Autodesk Fusion 360 part; units mm, degrees
note: some values were not read from the file. Chosen so that the rebuilt part matches the saved one: which bodies a step acts on.
(part 3 of 5)
sketch "スケッチ1 (13)" plane through (0, 0, 0) normal (0, 0, 1) x (1, 0, 0) in component "Stage2_Sun_Gear"
  line L0 (13.0702, -1.1985) -> (14.0365, -1.2871)
  line L1 (14.0365, -1.2871) -> (14.8505, -1.1753)
  line L2 (14.8505, -1.1753) -> (15.673, -0.8944)
  line L3 (15.673, -0.8944) -> (16.4928, -0.4881)
  line L4 (16.4928, -0.4881) -> (16.4928, 0.4881)
  line L5 (16.4928, 0.4881) -> (15.673, 0.8944)
  line L6 (15.673, 0.8944) -> (14.8505, 1.1753)
  line L7 (14.8505, 1.1753) -> (14.0365, 1.2871)
  line L8 (14.0365, 1.2871) -> (13.0702, 1.1985)
  line L9 (13.0702, 1.1985) -> (12.9634, 2.0532)
  line L10 (12.9634, 2.0532) -> (12.8008, 2.899)
  line L11 (12.8008, 2.899) -> (13.7473, 3.1134)
  line L12 (13.7473, 3.1134) -> (14.4868, 3.4713)
  line L13 (14.4868, 3.4713) -> (15.1822, 3.9926)
  line L14 (15.1822, 3.9926) -> (15.8364, 4.6323)
  line L15 (15.8364, 4.6323) -> (15.5347, 5.5607)
  line L16 (15.5347, 5.5607) -> (14.6295, 5.6938)
  line L17 (14.6295, 5.6938) -> (13.7605, 5.7068)
  line L18 (13.7605, 5.7068) -> (12.9518, 5.5617)
  line L19 (12.9518, 5.5617) -> (12.0601, 5.1788)
  line L20 (12.0601, 5.1788) -> (11.6945, 5.9586)
  line L21 (11.6945, 5.9586) -> (11.2785, 6.7128)
  line L22 (11.2785, 6.7128) -> (12.1123, 7.2091)
  line L23 (12.1123, 7.2091) -> (12.7051, 7.7781)
  line L24 (12.7051, 7.7781) -> (13.2054, 8.4888)
  line L25 (13.2054, 8.4888) -> (13.6298, 9.2993)
  line L26 (13.6298, 9.2993) -> (13.056, 10.0891)
  line L27 (13.056, 10.0891) -> (12.154, 9.9359)
  line L28 (12.154, 9.9359) -> (11.3235, 9.6797)
  line L29 (11.3235, 9.6797) -> (10.5992, 9.2918)
  line L30 (10.5992, 9.2918) -> (9.8695, 8.6521)
  line L31 (9.8695, 8.6521) -> (9.2808, 9.2808)
  line L32 (9.2808, 9.2808) -> (8.6521, 9.8695)
  line L33 (8.6521, 9.8695) -> (9.2918, 10.5992)
  line L34 (9.2918, 10.5992) -> (9.6797, 11.3235)
  line L35 (9.6797, 11.3235) -> (9.9359, 12.154)
  line L36 (9.9359, 12.154) -> (10.0891, 13.056)
  line L37 (10.0891, 13.056) -> (9.2993, 13.6298)
  line L38 (9.2993, 13.6298) -> (8.4888, 13.2054)
  line L39 (8.4888, 13.2054) -> (7.7781, 12.7051)
  line L40 (7.7781, 12.7051) -> (7.2091, 12.1123)
  line L41 (7.2091, 12.1123) -> (6.7128, 11.2785)
  line L42 (6.7128, 11.2785) -> (5.9586, 11.6945)
  line L43 (5.9586, 11.6945) -> (5.1788, 12.0601)
  line L44 (5.1788, 12.0601) -> (5.5617, 12.9518)
  line L45 (5.5617, 12.9518) -> (5.7068, 13.7605)
  line L46 (5.7068, 13.7605) -> (5.6938, 14.6295)
  line L47 (5.6938, 14.6295) -> (5.5607, 15.5347)
  line L48 (5.5607, 15.5347) -> (4.6323, 15.8364)
  line L49 (4.6323, 15.8364) -> (3.9926, 15.1822)
  line L50 (3.9926, 15.1822) -> (3.4713, 14.4868)
  line L51 (3.4713, 14.4868) -> (3.1134, 13.7473)
  line L52 (3.1134, 13.7473) -> (2.899, 12.8008)
  line L53 (2.899, 12.8008) -> (2.0532, 12.9634)
  line L54 (2.0532, 12.9634) -> (1.1985, 13.0702)
  line L55 (1.1985, 13.0702) -> (1.2871, 14.0365)
  line L56 (1.2871, 14.0365) -> (1.1753, 14.8505)
  line L57 (1.1753, 14.8505) -> (0.8944, 15.673)
  line L58 (0.8944, 15.673) -> (0.4881, 16.4928)
  line L59 (0.4881, 16.4928) -> (-0.4881, 16.4928)
  line L60 (-0.4881, 16.4928) -> (-0.8944, 15.673)
  line L61 (-0.8944, 15.673) -> (-1.1753, 14.8505)
  line L62 (-1.1753, 14.8505) -> (-1.2871, 14.0365)
  line L63 (-1.2871, 14.0365) -> (-1.1985, 13.0702)
  line L64 (-1.1985, 13.0702) -> (-2.0532, 12.9634)
  line L65 (-2.0532, 12.9634) -> (-2.899, 12.8008)
  line L66 (-2.899, 12.8008) -> (-3.1134, 13.7473)
  line L67 (-3.1134, 13.7473) -> (-3.4713, 14.4868)
  line L68 (-3.4713, 14.4868) -> (-3.9926, 15.1822)
  line L69 (-3.9926, 15.1822) -> (-4.6323, 15.8364)
  line L70 (-4.6323, 15.8364) -> (-5.5607, 15.5347)
  line L71 (-5.5607, 15.5347) -> (-5.6938, 14.6295)
  line L72 (-5.6938, 14.6295) -> (-5.7068, 13.7605)
  line L73 (-5.7068, 13.7605) -> (-5.5617, 12.9518)
  line L74 (-5.5617, 12.9518) -> (-5.1788, 12.0601)
  line L75 (-5.1788, 12.0601) -> (-5.9586, 11.6945)
  line L76 (-5.9586, 11.6945) -> (-6.7128, 11.2785)
  line L77 (-6.7128, 11.2785) -> (-7.2091, 12.1123)
  line L78 (-7.2091, 12.1123) -> (-7.7781, 12.7051)
  line L79 (-7.7781, 12.7051) -> (-8.4888, 13.2054)
  line L80 (-8.4888, 13.2054) -> (-9.2993, 13.6298)
  line L81 (-9.2993, 13.6298) -> (-10.0891, 13.056)
  line L82 (-10.0891, 13.056) -> (-9.9359, 12.154)
  line L83 (-9.9359, 12.154) -> (-9.6797, 11.3235)
  line L84 (-9.6797, 11.3235) -> (-9.2918, 10.5992)
  line L85 (-9.2918, 10.5992) -> (-8.6521, 9.8695)
  line L86 (-8.6521, 9.8695) -> (-9.2808, 9.2808)
  line L87 (-9.2808, 9.2808) -> (-9.8695, 8.6521)
  line L88 (-9.8695, 8.6521) -> (-10.5992, 9.2918)
  line L89 (-10.5992, 9.2918) -> (-11.3235, 9.6797)
  line L90 (-11.3235, 9.6797) -> (-12.154, 9.9359)
  line L91 (-12.154, 9.9359) -> (-13.056, 10.0891)
  line L92 (-13.056, 10.0891) -> (-13.6298, 9.2993)
  line L93 (-13.6298, 9.2993) -> (-13.2054, 8.4888)
  line L94 (-13.2054, 8.4888) -> (-12.7051, 7.7781)
  line L95 (-12.7051, 7.7781) -> (-12.1123, 7.2091)
  line L96 (-12.1123, 7.2091) -> (-11.2785, 6.7128)
  line L97 (-11.2785, 6.7128) -> (-11.6945, 5.9586)
  line L98 (-11.6945, 5.9586) -> (-12.0601, 5.1788)
  line L99 (-12.0601, 5.1788) -> (-12.9518, 5.5617)
  line L100 (-12.9518, 5.5617) -> (-13.7605, 5.7068)
  line L101 (-13.7605, 5.7068) -> (-14.6295, 5.6938)
  line L102 (-14.6295, 5.6938) -> (-15.5347, 5.5607)
  line L103 (-15.5347, 5.5607) -> (-15.8364, 4.6323)
  line L104 (-15.8364, 4.6323) -> (-15.1822, 3.9926)
  line L105 (-15.1822, 3.9926) -> (-14.4868, 3.4713)
  line L106 (-14.4868, 3.4713) -> (-13.7473, 3.1134)
  line L107 (-13.7473, 3.1134) -> (-12.8008, 2.899)
  line L108 (-12.8008, 2.899) -> (-12.9634, 2.0532)
  line L109 (-12.9634, 2.0532) -> (-13.0702, 1.1985)
  line L110 (-13.0702, 1.1985) -> (-14.0365, 1.2871)
  line L111 (-14.0365, 1.2871) -> (-14.8505, 1.1753)
  line L112 (-14.8505, 1.1753) -> (-15.673, 0.8944)
  line L113 (-15.673, 0.8944) -> (-16.4928, 0.4881)
  line L114 (-16.4928, 0.4881) -> (-16.4928, -0.4881)
  line L115 (-16.4928, -0.4881) -> (-15.673, -0.8944)
  line L116 (-15.673, -0.8944) -> (-14.8505, -1.1753)
  line L117 (-14.8505, -1.1753) -> (-14.0365, -1.2871)
  line L118 (-14.0365, -1.2871) -> (-13.0702, -1.1985)
  line L119 (-13.0702, -1.1985) -> (-12.9634, -2.0532)
  line L120 (-12.9634, -2.0532) -> (-12.8008, -2.899)
  line L121 (-12.8008, -2.899) -> (-13.7473, -3.1134)
  line L122 (-13.7473, -3.1134) -> (-14.4868, -3.4713)
  line L123 (-14.4868, -3.4713) -> (-15.1822, -3.9926)
  line L124 (-15.1822, -3.9926) -> (-15.8364, -4.6323)
  line L125 (-15.8364, -4.6323) -> (-15.5347, -5.5607)
  line L126 (-15.5347, -5.5607) -> (-14.6295, -5.6938)
  line L127 (-14.6295, -5.6938) -> (-13.7605, -5.7068)
  line L128 (-13.7605, -5.7068) -> (-12.9518, -5.5617)
  line L129 (-12.9518, -5.5617) -> (-12.0601, -5.1788)
  line L130 (-12.0601, -5.1788) -> (-11.6945, -5.9586)
  line L131 (-11.6945, -5.9586) -> (-11.2785, -6.7128)
  line L132 (-11.2785, -6.7128) -> (-12.1123, -7.2091)
  line L133 (-12.1123, -7.2091) -> (-12.7051, -7.7781)
  line L134 (-12.7051, -7.7781) -> (-13.2054, -8.4888)
  line L135 (-13.2054, -8.4888) -> (-13.6298, -9.2993)
  line L136 (-13.6298, -9.2993) -> (-13.056, -10.0891)
  line L137 (-13.056, -10.0891) -> (-12.154, -9.9359)
  line L138 (-12.154, -9.9359) -> (-11.3235, -9.6797)
  line L139 (-11.3235, -9.6797) -> (-10.5992, -9.2918)
  line L140 (-10.5992, -9.2918) -> (-9.8695, -8.6521)
  line L141 (-9.8695, -8.6521) -> (-9.2808, -9.2808)
  line L142 (-9.2808, -9.2808) -> (-8.6521, -9.8695)
  line L143 (-8.6521, -9.8695) -> (-9.2918, -10.5992)
  line L144 (-9.2918, -10.5992) -> (-9.6797, -11.3235)
  line L145 (-9.6797, -11.3235) -> (-9.9359, -12.154)
  line L146 (-9.9359, -12.154) -> (-10.0891, -13.056)
  line L147 (-10.0891, -13.056) -> (-9.2993, -13.6298)
  line L148 (-9.2993, -13.6298) -> (-8.4888, -13.2054)
  line L149 (-8.4888, -13.2054) -> (-7.7781, -12.7051)
  line L150 (-7.7781, -12.7051) -> (-7.2091, -12.1123)
  line L151 (-7.2091, -12.1123) -> (-6.7128, -11.2785)
  line L152 (-6.7128, -11.2785) -> (-5.9586, -11.6945)
  line L153 (-5.9586, -11.6945) -> (-5.1788, -12.0601)
  line L154 (-5.1788, -12.0601) -> (-5.5617, -12.9518)
  line L155 (-5.5617, -12.9518) -> (-5.7068, -13.7605)
  line L156 (-5.7068, -13.7605) -> (-5.6938, -14.6295)
  line L157 (-5.6938, -14.6295) -> (-5.5607, -15.5347)
  line L158 (-5.5607, -15.5347) -> (-4.6323, -15.8364)
  line L159 (-4.6323, -15.8364) -> (-3.9926, -15.1822)
  line L160 (-3.9926, -15.1822) -> (-3.4713, -14.4868)
  line L161 (-3.4713, -14.4868) -> (-3.1134, -13.7473)
  line L162 (-3.1134, -13.7473) -> (-2.899, -12.8008)
  line L163 (-2.899, -12.8008) -> (-2.0532, -12.9634)
  line L164 (-2.0532, -12.9634) -> (-1.1985, -13.0702)
  line L165 (-1.1985, -13.0702) -> (-1.2871, -14.0365)
  line L166 (-1.2871, -14.0365) -> (-1.1753, -14.8505)
  line L167 (-1.1753, -14.8505) -> (-0.8944, -15.673)
  line L168 (-0.8944, -15.673) -> (-0.4881, -16.4928)
  line L169 (-0.4881, -16.4928) -> (0.4881, -16.4928)
  line L170 (0.4881, -16.4928) -> (0.8944, -15.673)
  line L171 (0.8944, -15.673) -> (1.1753, -14.8505)
  line L172 (1.1753, -14.8505) -> (1.2871, -14.0365)
  line L173 (1.2871, -14.0365) -> (1.1985, -13.0702)
  line L174 (1.1985, -13.0702) -> (2.0532, -12.9634)
  line L175 (2.0532, -12.9634) -> (2.899, -12.8008)
  line L176 (2.899, -12.8008) -> (3.1134, -13.7473)
  line L177 (3.1134, -13.7473) -> (3.4713, -14.4868)
  line L178 (3.4713, -14.4868) -> (3.9926, -15.1822)
  line L179 (3.9926, -15.1822) -> (4.6323, -15.8364)
  line L180 (4.6323, -15.8364) -> (5.5607, -15.5347)
  line L181 (5.5607, -15.5347) -> (5.6938, -14.6295)
  line L182 (5.6938, -14.6295) -> (5.7068, -13.7605)
  line L183 (5.7068, -13.7605) -> (5.5617, -12.9518)
  line L184 (5.5617, -12.9518) -> (5.1788, -12.0601)
  line L185 (5.1788, -12.0601) -> (5.9586, -11.6945)
  line L186 (5.9586, -11.6945) -> (6.7128, -11.2785)
  line L187 (6.7128, -11.2785) -> (7.2091, -12.1123)
  line L188 (7.2091, -12.1123) -> (7.7781, -12.7051)
  line L189 (7.7781, -12.7051) -> (8.4888, -13.2054)
  line L190 (8.4888, -13.2054) -> (9.2993, -13.6298)
  line L191 (9.2993, -13.6298) -> (10.0891, -13.056)
  line L192 (10.0891, -13.056) -> (9.9359, -12.154)
  line L193 (9.9359, -12.154) -> (9.6797, -11.3235)
  line L194 (9.6797, -11.3235) -> (9.2918, -10.5992)
  line L195 (9.2918, -10.5992) -> (8.6521, -9.8695)
  line L196 (8.6521, -9.8695) -> (9.2808, -9.2808)
  line L197 (9.2808, -9.2808) -> (9.8695, -8.6521)
  line L198 (9.8695, -8.6521) -> (10.5992, -9.2918)
  line L199 (10.5992, -9.2918) -> (11.3235, -9.6797)
  line L200 (11.3235, -9.6797) -> (12.154, -9.9359)
  line L201 (12.154, -9.9359) -> (13.056, -10.0891)
  line L202 (13.056, -10.0891) -> (13.6298, -9.2993)
  line L203 (13.6298, -9.2993) -> (13.2054, -8.4888)
  line L204 (13.2054, -8.4888) -> (12.7051, -7.7781)
  line L205 (12.7051, -7.7781) -> (12.1123, -7.2091)
  line L206 (12.1123, -7.2091) -> (11.2785, -6.7128)
  line L207 (11.2785, -6.7128) -> (11.6945, -5.9586)
  line L208 (11.6945, -5.9586) -> (12.0601, -5.1788)
  line L209 (12.0601, -5.1788) -> (12.9518, -5.5617)
  line L210 (12.9518, -5.5617) -> (13.7605, -5.7068)
  line L211 (13.7605, -5.7068) -> (14.6295, -5.6938)
  line L212 (14.6295, -5.6938) -> (15.5347, -5.5607)
  line L213 (15.5347, -5.5607) -> (15.8364, -4.6323)
  line L214 (15.8364, -4.6323) -> (15.1822, -3.9926)
  line L215 (15.1822, -3.9926) -> (14.4868, -3.4713)
  line L216 (14.4868, -3.4713) -> (13.7473, -3.1134)
  line L217 (13.7473, -3.1134) -> (12.8008, -2.899)
  line L218 (12.8008, -2.899) -> (12.9634, -2.0532)
  line L219 (12.9634, -2.0532) -> (13.0702, -1.1985)
extrude "Stage2_Sun_Extrude" add sketch "スケッチ1 (13)" along normal blind 12 from surface at 74 separate body makes body 14 in component "Stage2_Sun_Gear"
sketch "スケッチ2 (13)" plane through (0, 0, 0) normal (0, 0, 1) x (1, 0, 0) in component "Stage2_Sun_Gear"
  circle A0 centre (0, 0) radius 12
extrude "Stage2_Sun_Hub_Lower_Extrude" add sketch "スケッチ2 (13)" along normal blind 3 from surface at 71 bodies 14 in component "Stage2_Sun_Gear"
sketch "スケッチ3 (12)" plane through (0, 0, 0) normal (0, 0, 1) x (1, 0, 0) in component "Stage2_Sun_Gear"
  circle A0 centre (0, 0) radius 12
extrude "Stage2_Sun_Hub_Upper_Extrude" add sketch "スケッチ3 (12)" along normal blind 3 from surface at 86 bodies 14 in component "Stage2_Sun_Gear"
sketch "スケッチ4 (12)" plane through (0, 0, 0) normal (0, 0, 1) x (1, 0, 0) in component "Stage2_Sun_Gear"
  circle A0 centre (0, 0) radius 8.1
extrude "Stage2_Sun_Bore_Cut" cut sketch "スケッチ4 (12)" along normal blind 20 from surface at 70 bodies 14 in component "Stage2_Sun_Gear"
sketch "スケッチ1 (14)" plane through (0, 0, 0) normal (0, 0, 1) x (1, 0, 0) in component "Stage2_Planet_Gear_A"
  line L0 (17.2782, 3.2284) -> (16.3377, 3.4671)
  line L1 (16.3377, 3.4671) -> (15.5162, 3.4839)
  line L2 (15.5162, 3.4839) -> (14.6599, 3.3351)
  line L3 (14.6599, 3.3351) -> (13.7866, 3.0621)
  line L4 (13.7866, 3.0621) -> (13.6339, 2.098)
  line L5 (13.6339, 2.098) -> (14.3801, 1.5685)
  line L6 (14.3801, 1.5685) -> (15.1485, 1.1623)
  line L7 (15.1485, 1.1623) -> (15.935, 0.9245)
  line L8 (15.935, 0.9245) -> (16.9033, 0.8608)
  line L9 (16.9033, 0.8608) -> (16.875, 0)
  line L10 (16.875, 0) -> (16.9033, -0.8608)
  line L11 (16.9033, -0.8608) -> (15.935, -0.9245)
  line L12 (15.935, -0.9245) -> (15.1485, -1.1623)
  line L13 (15.1485, -1.1623) -> (14.3801, -1.5685)
  line L14 (14.3801, -1.5685) -> (13.6339, -2.098)
  line L15 (13.6339, -2.098) -> (13.7866, -3.0621)
  line L16 (13.7866, -3.0621) -> (14.6599, -3.3351)
  line L17 (14.6599, -3.3351) -> (15.5162, -3.4839)
  line L18 (15.5162, -3.4839) -> (16.3377, -3.4671)
  line L19 (16.3377, -3.4671) -> (17.2782, -3.2284)
  line L20 (17.2782, -3.2284) -> (17.5174, -4.0558)
  line L21 (17.5174, -4.0558) -> (17.8103, -4.8658)
  line L22 (17.8103, -4.8658) -> (16.909, -5.2256)
  line L23 (16.909, -5.2256) -> (16.2346, -5.6948)
  line L24 (16.2346, -5.6948) -> (15.6293, -6.3185)
  line L25 (15.6293, -6.3185) -> (15.0832, -7.0527)
  line L26 (15.0832, -7.0527) -> (15.5264, -7.9225)
  line L27 (15.5264, -7.9225) -> (16.4413, -7.9123)
  line L28 (16.4413, -7.9123) -> (17.3017, -7.7891)
  line L29 (17.3017, -7.7891) -> (18.0777, -7.5193)
  line L30 (18.0777, -7.5193) -> (18.8985, -7.0016)
  line L31 (18.8985, -7.0016) -> (19.3817, -7.7147)
  line L32 (19.3817, -7.7147) -> (19.9105, -8.3945)
  line L33 (19.9105, -8.3945) -> (19.1645, -9.0152)
  line L34 (19.1645, -9.0152) -> (18.6681, -9.6699)
  line L35 (18.6681, -9.6699) -> (18.2851, -10.4501)
  line L36 (18.2851, -10.4501) -> (17.9927, -11.317)
  line L37 (17.9927, -11.317) -> (18.683, -12.0073)
  line L38 (18.683, -12.0073) -> (19.5499, -11.7149)
  line L39 (19.5499, -11.7149) -> (20.3301, -11.3319)
  line L40 (20.3301, -11.3319) -> (20.9848, -10.8355)
  line L41 (20.9848, -10.8355) -> (21.6055, -10.0895)
  line L42 (21.6055, -10.0895) -> (22.2853, -10.6183)
  line L43 (22.2853, -10.6183) -> (22.9984, -11.1015)
  line L44 (22.9984, -11.1015) -> (22.4807, -11.9223)
  line L45 (22.4807, -11.9223) -> (22.2109, -12.6983)
  line L46 (22.2109, -12.6983) -> (22.0877, -13.5587)
  line L47 (22.0877, -13.5587) -> (22.0775, -14.4736)
  line L48 (22.0775, -14.4736) -> (22.9473, -14.9168)
  line L49 (22.9473, -14.9168) -> (23.6815, -14.3707)
  line L50 (23.6815, -14.3707) -> (24.3052, -13.7654)
  line L51 (24.3052, -13.7654) -> (24.7744, -13.091)
  line L52 (24.7744, -13.091) -> (25.1342, -12.1897)
  line L53 (25.1342, -12.1897) -> (25.9442, -12.4826)
  line L54 (25.9442, -12.4826) -> (26.7716, -12.7218)
  line L55 (26.7716, -12.7218) -> (26.5329, -13.6623)
  line L56 (26.5329, -13.6623) -> (26.5161, -14.4838)
  line L57 (26.5161, -14.4838) -> (26.6649, -15.3401)
  line L58 (26.6649, -15.3401) -> (26.9379, -16.2134)
  line L59 (26.9379, -16.2134) -> (27.902, -16.3661)
  line L60 (27.902, -16.3661) -> (28.4315, -15.6199)
  line L61 (28.4315, -15.6199) -> (28.8377, -14.8515)
  line L62 (28.8377, -14.8515) -> (29.0755, -14.065)
  line L63 (29.0755, -14.065) -> (29.1392, -13.0967)
  line L64 (29.1392, -13.0967) -> (30, -13.125)
  line L65 (30, -13.125) -> (30.8608, -13.0967)
  line L66 (30.8608, -13.0967) -> (30.9245, -14.065)
  line L67 (30.9245, -14.065) -> (31.1623, -14.8515)
  line L68 (31.1623, -14.8515) -> (31.5685, -15.6199)
  line L69 (31.5685, -15.6199) -> (32.098, -16.3661)
  line L70 (32.098, -16.3661) -> (33.0621, -16.2134)
  line L71 (33.0621, -16.2134) -> (33.3351, -15.3401)
  line L72 (33.3351, -15.3401) -> (33.4839, -14.4838)
  line L73 (33.4839, -14.4838) -> (33.4671, -13.6623)
  line L74 (33.4671, -13.6623) -> (33.2284, -12.7218)
  line L75 (33.2284, -12.7218) -> (34.0558, -12.4826)
  line L76 (34.0558, -12.4826) -> (34.8658, -12.1897)
  line L77 (34.8658, -12.1897) -> (35.2256, -13.091)
  line L78 (35.2256, -13.091) -> (35.6948, -13.7654)
  line L79 (35.6948, -13.7654) -> (36.3185, -14.3707)
  line L80 (36.3185, -14.3707) -> (37.0527, -14.9168)
  line L81 (37.0527, -14.9168) -> (37.9225, -14.4736)
  line L82 (37.9225, -14.4736) -> (37.9123, -13.5587)
  line L83 (37.9123, -13.5587) -> (37.7891, -12.6983)
  line L84 (37.7891, -12.6983) -> (37.5193, -11.9223)
  line L85 (37.5193, -11.9223) -> (37.0016, -11.1015)
  line L86 (37.0016, -11.1015) -> (37.7147, -10.6183)
  line L87 (37.7147, -10.6183) -> (38.3945, -10.0895)
  line L88 (38.3945, -10.0895) -> (39.0152, -10.8355)
  line L89 (39.0152, -10.8355) -> (39.6699, -11.3319)
  line L90 (39.6699, -11.3319) -> (40.4501, -11.7149)
  line L91 (40.4501, -11.7149) -> (41.317, -12.0073)
  line L92 (41.317, -12.0073) -> (42.0073, -11.317)
  line L93 (42.0073, -11.317) -> (41.7149, -10.4501)
  line L94 (41.7149, -10.4501) -> (41.3319, -9.6699)
  line L95 (41.3319, -9.6699) -> (40.8355, -9.0152)
  line L96 (40.8355, -9.0152) -> (40.0895, -8.3945)
  line L97 (40.0895, -8.3945) -> (40.6183, -7.7147)
  line L98 (40.6183, -7.7147) -> (41.1015, -7.0016)
  line L99 (41.1015, -7.0016) -> (41.9223, -7.5193)
  line L100 (41.9223, -7.5193) -> (42.6983, -7.7891)
  line L101 (42.6983, -7.7891) -> (43.5587, -7.9123)
  line L102 (43.5587, -7.9123) -> (44.4736, -7.9225)
  line L103 (44.4736, -7.9225) -> (44.9168, -7.0527)
  line L104 (44.9168, -7.0527) -> (44.3707, -6.3185)
  line L105 (44.3707, -6.3185) -> (43.7654, -5.6948)
  line L106 (43.7654, -5.6948) -> (43.091, -5.2256)
  line L107 (43.091, -5.2256) -> (42.1897, -4.8658)
  line L108 (42.1897, -4.8658) -> (42.4826, -4.0558)
  line L109 (42.4826, -4.0558) -> (42.7218, -3.2284)
  line L110 (42.7218, -3.2284) -> (43.6623, -3.4671)
  line L111 (43.6623, -3.4671) -> (44.4838, -3.4839)
  line L112 (44.4838, -3.4839) -> (45.3401, -3.3351)
  line L113 (45.3401, -3.3351) -> (46.2134, -3.0621)
  line L114 (46.2134, -3.0621) -> (46.3661, -2.098)
  line L115 (46.3661, -2.098) -> (45.6199, -1.5685)
  line L116 (45.6199, -1.5685) -> (44.8515, -1.1623)
  line L117 (44.8515, -1.1623) -> (44.065, -0.9245)
  line L118 (44.065, -0.9245) -> (43.0967, -0.8608)
  line L119 (43.0967, -0.8608) -> (43.125, 0)
  line L120 (43.125, 0) -> (43.0967, 0.8608)
  line L121 (43.0967, 0.8608) -> (44.065, 0.9245)
  line L122 (44.065, 0.9245) -> (44.8515, 1.1623)
  line L123 (44.8515, 1.1623) -> (45.6199, 1.5685)
  line L124 (45.6199, 1.5685) -> (46.3661, 2.098)
  line L125 (46.3661, 2.098) -> (46.2134, 3.0621)
  line L126 (46.2134, 3.0621) -> (45.3401, 3.3351)
  line L127 (45.3401, 3.3351) -> (44.4838, 3.4839)
  line L128 (44.4838, 3.4839) -> (43.6623, 3.4671)
  line L129 (43.6623, 3.4671) -> (42.7218, 3.2284)
  line L130 (42.7218, 3.2284) -> (42.4826, 4.0558)
  line L131 (42.4826, 4.0558) -> (42.1897, 4.8658)
  line L132 (42.1897, 4.8658) -> (43.091, 5.2256)
  line L133 (43.091, 5.2256) -> (43.7654, 5.6948)
  line L134 (43.7654, 5.6948) -> (44.3707, 6.3185)
  line L135 (44.3707, 6.3185) -> (44.9168, 7.0527)
  line L136 (44.9168, 7.0527) -> (44.4736, 7.9225)
  line L137 (44.4736, 7.9225) -> (43.5587, 7.9123)
  line L138 (43.5587, 7.9123) -> (42.6983, 7.7891)
  line L139 (42.6983, 7.7891) -> (41.9223, 7.5193)
  line L140 (41.9223, 7.5193) -> (41.1015, 7.0016)
  line L141 (41.1015, 7.0016) -> (40.6183, 7.7147)
  line L142 (40.6183, 7.7147) -> (40.0895, 8.3945)
  line L143 (40.0895, 8.3945) -> (40.8355, 9.0152)
  line L144 (40.8355, 9.0152) -> (41.3319, 9.6699)
  line L145 (41.3319, 9.6699) -> (41.7149, 10.4501)
  line L146 (41.7149, 10.4501) -> (42.0073, 11.317)
  line L147 (42.0073, 11.317) -> (41.317, 12.0073)
  line L148 (41.317, 12.0073) -> (40.4501, 11.7149)
  line L149 (40.4501, 11.7149) -> (39.6699, 11.3319)
  line L150 (39.6699, 11.3319) -> (39.0152, 10.8355)
  line L151 (39.0152, 10.8355) -> (38.3945, 10.0895)
  line L152 (38.3945, 10.0895) -> (37.7147, 10.6183)
  line L153 (37.7147, 10.6183) -> (37.0016, 11.1015)
  line L154 (37.0016, 11.1015) -> (37.5193, 11.9223)
  line L155 (37.5193, 11.9223) -> (37.7891, 12.6983)
  line L156 (37.7891, 12.6983) -> (37.9123, 13.5587)
  line L157 (37.9123, 13.5587) -> (37.9225, 14.4736)
  line L158 (37.9225, 14.4736) -> (37.0527, 14.9168)
  line L159 (37.0527, 14.9168) -> (36.3185, 14.3707)
  line L160 (36.3185, 14.3707) -> (35.6948, 13.7654)
  line L161 (35.6948, 13.7654) -> (35.2256, 13.091)
  line L162 (35.2256, 13.091) -> (34.8658, 12.1897)
  line L163 (34.8658, 12.1897) -> (34.0558, 12.4826)
  line L164 (34.0558, 12.4826) -> (33.2284, 12.7218)
  line L165 (33.2284, 12.7218) -> (33.4671, 13.6623)
  line L166 (33.4671, 13.6623) -> (33.4839, 14.4838)
  line L167 (33.4839, 14.4838) -> (33.3351, 15.3401)
  line L168 (33.3351, 15.3401) -> (33.0621, 16.2134)
  line L169 (33.0621, 16.2134) -> (32.098, 16.3661)
  line L170 (32.098, 16.3661) -> (31.5685, 15.6199)
  line L171 (31.5685, 15.6199) -> (31.1623, 14.8515)
  line L172 (31.1623, 14.8515) -> (30.9245, 14.065)
  line L173 (30.9245, 14.065) -> (30.8608, 13.0967)
  line L174 (30.8608, 13.0967) -> (30, 13.125)
  line L175 (30, 13.125) -> (29.1392, 13.0967)
  line L176 (29.1392, 13.0967) -> (29.0755, 14.065)
  line L177 (29.0755, 14.065) -> (28.8377, 14.8515)
  line L178 (28.8377, 14.8515) -> (28.4315, 15.6199)
  line L179 (28.4315, 15.6199) -> (27.902, 16.3661)
  line L180 (27.902, 16.3661) -> (26.9379, 16.2134)
  line L181 (26.9379, 16.2134) -> (26.6649, 15.3401)
  line L182 (26.6649, 15.3401) -> (26.5161, 14.4838)
  line L183 (26.5161, 14.4838) -> (26.5329, 13.6623)
  line L184 (26.5329, 13.6623) -> (26.7716, 12.7218)
  line L185 (26.7716, 12.7218) -> (25.9442, 12.4826)
  line L186 (25.9442, 12.4826) -> (25.1342, 12.1897)
  line L187 (25.1342, 12.1897) -> (24.7744, 13.091)
  line L188 (24.7744, 13.091) -> (24.3052, 13.7654)
  line L189 (24.3052, 13.7654) -> (23.6815, 14.3707)
  line L190 (23.6815, 14.3707) -> (22.9473, 14.9168)
  line L191 (22.9473, 14.9168) -> (22.0775, 14.4736)
  line L192 (22.0775, 14.4736) -> (22.0877, 13.5587)
  line L193 (22.0877, 13.5587) -> (22.2109, 12.6983)
  line L194 (22.2109, 12.6983) -> (22.4807, 11.9223)
  line L195 (22.4807, 11.9223) -> (22.9984, 11.1015)
  line L196 (22.9984, 11.1015) -> (22.2853, 10.6183)
  line L197 (22.2853, 10.6183) -> (21.6055, 10.0895)
  line L198 (21.6055, 10.0895) -> (20.9848, 10.8355)
  line L199 (20.9848, 10.8355) -> (20.3301, 11.3319)
  line L200 (20.3301, 11.3319) -> (19.5499, 11.7149)
  line L201 (19.5499, 11.7149) -> (18.683, 12.0073)
  line L202 (18.683, 12.0073) -> (17.9927, 11.317)
  line L203 (17.9927, 11.317) -> (18.2851, 10.4501)
  line L204 (18.2851, 10.4501) -> (18.6681, 9.6699)
  line L205 (18.6681, 9.6699) -> (19.1645, 9.0152)
  line L206 (19.1645, 9.0152) -> (19.9105, 8.3945)
  line L207 (19.9105, 8.3945) -> (19.3817, 7.7147)
  line L208 (19.3817, 7.7147) -> (18.8985, 7.0016)
  line L209 (18.8985, 7.0016) -> (18.0777, 7.5193)
  line L210 (18.0777, 7.5193) -> (17.3017, 7.7891)
  line L211 (17.3017, 7.7891) -> (16.4413, 7.9123)
  line L212 (16.4413, 7.9123) -> (15.5264, 7.9225)
  line L213 (15.5264, 7.9225) -> (15.0832, 7.0527)
  line L214 (15.0832, 7.0527) -> (15.6293, 6.3185)
  line L215 (15.6293, 6.3185) -> (16.2346, 5.6948)
  line L216 (16.2346, 5.6948) -> (16.909, 5.2256)
  line L217 (16.909, 5.2256) -> (17.8103, 4.8658)
  line L218 (17.8103, 4.8658) -> (17.5174, 4.0558)
  line L219 (17.5174, 4.0558) -> (17.2782, 3.2284)
extrude "Stage2_Planet_A_Extrude" add sketch "スケッチ1 (14)" along normal blind 12 from surface at 74 separate body makes body 15 in component "Stage2_Planet_Gear_A"
sketch "スケッチ2 (14)" plane through (0, 0, 0) normal (0, 0, 1) x (1, 0, 0) in component "Stage2_Planet_Gear_A"
  circle A0 centre (30, 0) radius 9
extrude "Stage2_Planet_A_Hub_Lower_Extrude" add sketch "スケッチ2 (14)" along normal blind 3 from surface at 71 bodies 15 in component "Stage2_Planet_Gear_A"
sketch "スケッチ3 (13)" plane through (0, 0, 0) normal (0, 0, 1) x (1, 0, 0) in component "Stage2_Planet_Gear_A"
  circle A0 centre (30, 0) radius 9
extrude "Stage2_Planet_A_Hub_Upper_Extrude" add sketch "スケッチ3 (13)" along normal blind 3 from surface at 86 bodies 15 in component "Stage2_Planet_Gear_A"
sketch "スケッチ4 (13)" plane through (0, 0, 0) normal (0, 0, 1) x (1, 0, 0) in component "Stage2_Planet_Gear_A"
  circle A0 centre (30, 0) radius 4.3
extrude "Stage2_Planet_A_Bore_Cut" cut sketch "スケッチ4 (13)" along normal blind 20 from surface at 70 bodies 15 in component "Stage2_Planet_Gear_A"
sketch "スケッチ1 (15)" plane through (0, 0, 0) normal (0, 0, 1) x (1, 0, 0) in component "Stage2_Planet_Gear_B"
  line L0 (-12.7218, 33.2284) -> (-13.6623, 33.4671)
  line L1 (-13.6623, 33.4671) -> (-14.4838, 33.4839)
  line L2 (-14.4838, 33.4839) -> (-15.3401, 33.3351)
  line L3 (-15.3401, 33.3351) -> (-16.2134, 33.0621)
  line L4 (-16.2134, 33.0621) -> (-16.3661, 32.098)
  line L5 (-16.3661, 32.098) -> (-15.6199, 31.5685)
  line L6 (-15.6199, 31.5685) -> (-14.8515, 31.1623)
  line L7 (-14.8515, 31.1623) -> (-14.065, 30.9245)
  line L8 (-14.065, 30.9245) -> (-13.0967, 30.8608)
  line L9 (-13.0967, 30.8608) -> (-13.125, 30)
  line L10 (-13.125, 30) -> (-13.0967, 29.1392)
  line L11 (-13.0967, 29.1392) -> (-14.065, 29.0755)
  line L12 (-14.065, 29.0755) -> (-14.8515, 28.8377)
  line L13 (-14.8515, 28.8377) -> (-15.6199, 28.4315)
  line L14 (-15.6199, 28.4315) -> (-16.3661, 27.902)
  line L15 (-16.3661, 27.902) -> (-16.2134, 26.9379)
  line L16 (-16.2134, 26.9379) -> (-15.3401, 26.6649)
  line L17 (-15.3401, 26.6649) -> (-14.4838, 26.5161)
  line L18 (-14.4838, 26.5161) -> (-13.6623, 26.5329)
  line L19 (-13.6623, 26.5329) -> (-12.7218, 26.7716)
  line L20 (-12.7218, 26.7716) -> (-12.4826, 25.9442)
  line L21 (-12.4826, 25.9442) -> (-12.1897, 25.1342)
  line L22 (-12.1897, 25.1342) -> (-13.091, 24.7744)
  line L23 (-13.091, 24.7744) -> (-13.7654, 24.3052)
  line L24 (-13.7654, 24.3052) -> (-14.3707, 23.6815)
  line L25 (-14.3707, 23.6815) -> (-14.9168, 22.9473)
  line L26 (-14.9168, 22.9473) -> (-14.4736, 22.0775)
  line L27 (-14.4736, 22.0775) -> (-13.5587, 22.0877)
  line L28 (-13.5587, 22.0877) -> (-12.6983, 22.2109)
  line L29 (-12.6983, 22.2109) -> (-11.9223, 22.4807)
  line L30 (-11.9223, 22.4807) -> (-11.1015, 22.9984)
  line L31 (-11.1015, 22.9984) -> (-10.6183, 22.2853)
  line L32 (-10.6183, 22.2853) -> (-10.0895, 21.6055)
  line L33 (-10.0895, 21.6055) -> (-10.8355, 20.9848)
  line L34 (-10.8355, 20.9848) -> (-11.3319, 20.3301)
  line L35 (-11.3319, 20.3301) -> (-11.7149, 19.5499)
  line L36 (-11.7149, 19.5499) -> (-12.0073, 18.683)
  line L37 (-12.0073, 18.683) -> (-11.317, 17.9927)
  line L38 (-11.317, 17.9927) -> (-10.4501, 18.2851)
  line L39 (-10.4501, 18.2851) -> (-9.6699, 18.6681)
  line L40 (-9.6699, 18.6681) -> (-9.0152, 19.1645)
  line L41 (-9.0152, 19.1645) -> (-8.3945, 19.9105)
  line L42 (-8.3945, 19.9105) -> (-7.7147, 19.3817)
  line L43 (-7.7147, 19.3817) -> (-7.0016, 18.8985)
  line L44 (-7.0016, 18.8985) -> (-7.5193, 18.0777)
  line L45 (-7.5193, 18.0777) -> (-7.7891, 17.3017)
  line L46 (-7.7891, 17.3017) -> (-7.9123, 16.4413)
  line L47 (-7.9123, 16.4413) -> (-7.9225, 15.5264)
  line L48 (-7.9225, 15.5264) -> (-7.0527, 15.0832)
  line L49 (-7.0527, 15.0832) -> (-6.3185, 15.6293)
  line L50 (-6.3185, 15.6293) -> (-5.6948, 16.2346)
  line L51 (-5.6948, 16.2346) -> (-5.2256, 16.909)
  line L52 (-5.2256, 16.909) -> (-4.8658, 17.8103)
  line L53 (-4.8658, 17.8103) -> (-4.0558, 17.5174)
  line L54 (-4.0558, 17.5174) -> (-3.2284, 17.2782)
  line L55 (-3.2284, 17.2782) -> (-3.4671, 16.3377)
  line L56 (-3.4671, 16.3377) -> (-3.4839, 15.5162)
  line L57 (-3.4839, 15.5162) -> (-3.3351, 14.6599)
  line L58 (-3.3351, 14.6599) -> (-3.0621, 13.7866)
  line L59 (-3.0621, 13.7866) -> (-2.098, 13.6339)
  line L60 (-2.098, 13.6339) -> (-1.5685, 14.3801)
  line L61 (-1.5685, 14.3801) -> (-1.1623, 15.1485)
  line L62 (-1.1623, 15.1485) -> (-0.9245, 15.935)
  line L63 (-0.9245, 15.935) -> (-0.8608, 16.9033)
  line L64 (-0.8608, 16.9033) -> (0, 16.875)
  line L65 (0, 16.875) -> (0.8608, 16.9033)
  line L66 (0.8608, 16.9033) -> (0.9245, 15.935)
  line L67 (0.9245, 15.935) -> (1.1623, 15.1485)
  line L68 (1.1623, 15.1485) -> (1.5685, 14.3801)
  line L69 (1.5685, 14.3801) -> (2.098, 13.6339)
  line L70 (2.098, 13.6339) -> (3.0621, 13.7866)
  line L71 (3.0621, 13.7866) -> (3.3351, 14.6599)
  line L72 (3.3351, 14.6599) -> (3.4839, 15.5162)
  line L73 (3.4839, 15.5162) -> (3.4671, 16.3377)
  line L74 (3.4671, 16.3377) -> (3.2284, 17.2782)
  line L75 (3.2284, 17.2782) -> (4.0558, 17.5174)
  line L76 (4.0558, 17.5174) -> (4.8658, 17.8103)
  line L77 (4.8658, 17.8103) -> (5.2256, 16.909)
  line L78 (5.2256, 16.909) -> (5.6948, 16.2346)
  line L79 (5.6948, 16.2346) -> (6.3185, 15.6293)
  line L80 (6.3185, 15.6293) -> (7.0527, 15.0832)
  line L81 (7.0527, 15.0832) -> (7.9225, 15.5264)
  line L82 (7.9225, 15.5264) -> (7.9123, 16.4413)
  line L83 (7.9123, 16.4413) -> (7.7891, 17.3017)
  line L84 (7.7891, 17.3017) -> (7.5193, 18.0777)
  line L85 (7.5193, 18.0777) -> (7.0016, 18.8985)
  line L86 (7.0016, 18.8985) -> (7.7147, 19.3817)
  line L87 (7.7147, 19.3817) -> (8.3945, 19.9105)
  line L88 (8.3945, 19.9105) -> (9.0152, 19.1645)
  line L89 (9.0152, 19.1645) -> (9.6699, 18.6681)
  line L90 (9.6699, 18.6681) -> (10.4501, 18.2851)
  line L91 (10.4501, 18.2851) -> (11.317, 17.9927)
  line L92 (11.317, 17.9927) -> (12.0073, 18.683)
  line L93 (12.0073, 18.683) -> (11.7149, 19.5499)
  line L94 (11.7149, 19.5499) -> (11.3319, 20.3301)
  line L95 (11.3319, 20.3301) -> (10.8355, 20.9848)
  line L96 (10.8355, 20.9848) -> (10.0895, 21.6055)
  line L97 (10.0895, 21.6055) -> (10.6183, 22.2853)
  line L98 (10.6183, 22.2853) -> (11.1015, 22.9984)
  line L99 (11.1015, 22.9984) -> (11.9223, 22.4807)
  line L100 (11.9223, 22.4807) -> (12.6983, 22.2109)
  line L101 (12.6983, 22.2109) -> (13.5587, 22.0877)
  line L102 (13.5587, 22.0877) -> (14.4736, 22.0775)
  line L103 (14.4736, 22.0775) -> (14.9168, 22.9473)
  line L104 (14.9168, 22.9473) -> (14.3707, 23.6815)
  line L105 (14.3707, 23.6815) -> (13.7654, 24.3052)
  line L106 (13.7654, 24.3052) -> (13.091, 24.7744)
  line L107 (13.091, 24.7744) -> (12.1897, 25.1342)
  line L108 (12.1897, 25.1342) -> (12.4826, 25.9442)
  line L109 (12.4826, 25.9442) -> (12.7218, 26.7716)
  line L110 (12.7218, 26.7716) -> (13.6623, 26.5329)
  line L111 (13.6623, 26.5329) -> (14.4838, 26.5161)
  line L112 (14.4838, 26.5161) -> (15.3401, 26.6649)
  line L113 (15.3401, 26.6649) -> (16.2134, 26.9379)
  line L114 (16.2134, 26.9379) -> (16.3661, 27.902)
  line L115 (16.3661, 27.902) -> (15.6199, 28.4315)
  line L116 (15.6199, 28.4315) -> (14.8515, 28.8377)
  line L117 (14.8515, 28.8377) -> (14.065, 29.0755)
  line L118 (14.065, 29.0755) -> (13.0967, 29.1392)
  line L119 (13.0967, 29.1392) -> (13.125, 30)
  line L120 (13.125, 30) -> (13.0967, 30.8608)
  line L121 (13.0967, 30.8608) -> (14.065, 30.9245)
  line L122 (14.065, 30.9245) -> (14.8515, 31.1623)
  line L123 (14.8515, 31.1623) -> (15.6199, 31.5685)
  line L124 (15.6199, 31.5685) -> (16.3661, 32.098)
  line L125 (16.3661, 32.098) -> (16.2134, 33.0621)
  line L126 (16.2134, 33.0621) -> (15.3401, 33.3351)
  line L127 (15.3401, 33.3351) -> (14.4838, 33.4839)
  line L128 (14.4838, 33.4839) -> (13.6623, 33.4671)
  line L129 (13.6623, 33.4671) -> (12.7218, 33.2284)
  line L130 (12.7218, 33.2284) -> (12.4826, 34.0558)
  line L131 (12.4826, 34.0558) -> (12.1897, 34.8658)
  line L132 (12.1897, 34.8658) -> (13.091, 35.2256)
  line L133 (13.091, 35.2256) -> (13.7654, 35.6948)
  line L134 (13.7654, 35.6948) -> (14.3707, 36.3185)
  line L135 (14.3707, 36.3185) -> (14.9168, 37.0527)
  line L136 (14.9168, 37.0527) -> (14.4736, 37.9225)
  line L137 (14.4736, 37.9225) -> (13.5587, 37.9123)
  line L138 (13.5587, 37.9123) -> (12.6983, 37.7891)
  line L139 (12.6983, 37.7891) -> (11.9223, 37.5193)
  line L140 (11.9223, 37.5193) -> (11.1015, 37.0016)
  line L141 (11.1015, 37.0016) -> (10.6183, 37.7147)
  line L142 (10.6183, 37.7147) -> (10.0895, 38.3945)
  line L143 (10.0895, 38.3945) -> (10.8355, 39.0152)
  line L144 (10.8355, 39.0152) -> (11.3319, 39.6699)
  line L145 (11.3319, 39.6699) -> (11.7149, 40.4501)
  line L146 (11.7149, 40.4501) -> (12.0073, 41.317)
  line L147 (12.0073, 41.317) -> (11.317, 42.0073)
  line L148 (11.317, 42.0073) -> (10.4501, 41.7149)
  line L149 (10.4501, 41.7149) -> (9.6699, 41.3319)
  line L150 (9.6699, 41.3319) -> (9.0152, 40.8355)
  line L151 (9.0152, 40.8355) -> (8.3945, 40.0895)
  line L152 (8.3945, 40.0895) -> (7.7147, 40.6183)
  line L153 (7.7147, 40.6183) -> (7.0016, 41.1015)
  line L154 (7.0016, 41.1015) -> (7.5193, 41.9223)
  line L155 (7.5193, 41.9223) -> (7.7891, 42.6983)
  line L156 (7.7891, 42.6983) -> (7.9123, 43.5587)
  line L157 (7.9123, 43.5587) -> (7.9225, 44.4736)
  line L158 (7.9225, 44.4736) -> (7.0527, 44.9168)
  line L159 (7.0527, 44.9168) -> (6.3185, 44.3707)
  line L160 (6.3185, 44.3707) -> (5.6948, 43.7654)
  line L161 (5.6948, 43.7654) -> (5.2256, 43.091)
  line L162 (5.2256, 43.091) -> (4.8658, 42.1897)
  line L163 (4.8658, 42.1897) -> (4.0558, 42.4826)
  line L164 (4.0558, 42.4826) -> (3.2284, 42.7218)
  line L165 (3.2284, 42.7218) -> (3.4671, 43.6623)
  line L166 (3.4671, 43.6623) -> (3.4839, 44.4838)
  line L167 (3.4839, 44.4838) -> (3.3351, 45.3401)
  line L168 (3.3351, 45.3401) -> (3.0621, 46.2134)
  line L169 (3.0621, 46.2134) -> (2.098, 46.3661)
  line L170 (2.098, 46.3661) -> (1.5685, 45.6199)
  line L171 (1.5685, 45.6199) -> (1.1623, 44.8515)
  line L172 (1.1623, 44.8515) -> (0.9245, 44.065)
  line L173 (0.9245, 44.065) -> (0.8608, 43.0967)
  line L174 (0.8608, 43.0967) -> (0, 43.125)
  line L175 (0, 43.125) -> (-0.8608, 43.0967)
  line L176 (-0.8608, 43.0967) -> (-0.9245, 44.065)
  line L177 (-0.9245, 44.065) -> (-1.1623, 44.8515)
  line L178 (-1.1623, 44.8515) -> (-1.5685, 45.6199)
  line L179 (-1.5685, 45.6199) -> (-2.098, 46.3661)
  line L180 (-2.098, 46.3661) -> (-3.0621, 46.2134)
  line L181 (-3.0621, 46.2134) -> (-3.3351, 45.3401)
  line L182 (-3.3351, 45.3401) -> (-3.4839, 44.4838)
  line L183 (-3.4839, 44.4838) -> (-3.4671, 43.6623)
  line L184 (-3.4671, 43.6623) -> (-3.2284, 42.7218)
  line L185 (-3.2284, 42.7218) -> (-4.0558, 42.4826)
  line L186 (-4.0558, 42.4826) -> (-4.8658, 42.1897)
  line L187 (-4.8658, 42.1897) -> (-5.2256, 43.091)
  line L188 (-5.2256, 43.091) -> (-5.6948, 43.7654)
  line L189 (-5.6948, 43.7654) -> (-6.3185, 44.3707)
  line L190 (-6.3185, 44.3707) -> (-7.0527, 44.9168)
  line L191 (-7.0527, 44.9168) -> (-7.9225, 44.4736)
  line L192 (-7.9225, 44.4736) -> (-7.9123, 43.5587)
  line L193 (-7.9123, 43.5587) -> (-7.7891, 42.6983)
  line L194 (-7.7891, 42.6983) -> (-7.5193, 41.9223)
  line L195 (-7.5193, 41.9223) -> (-7.0016, 41.1015)
  line L196 (-7.0016, 41.1015) -> (-7.7147, 40.6183)
  line L197 (-7.7147, 40.6183) -> (-8.3945, 40.0895)
  line L198 (-8.3945, 40.0895) -> (-9.0152, 40.8355)
  line L199 (-9.0152, 40.8355) -> (-9.6699, 41.3319)
  line L200 (-9.6699, 41.3319) -> (-10.4501, 41.7149)
  line L201 (-10.4501, 41.7149) -> (-11.317, 42.0073)
  line L202 (-11.317, 42.0073) -> (-12.0073, 41.317)
  line L203 (-12.0073, 41.317) -> (-11.7149, 40.4501)
  line L204 (-11.7149, 40.4501) -> (-11.3319, 39.6699)
  line L205 (-11.3319, 39.6699) -> (-10.8355, 39.0152)
  line L206 (-10.8355, 39.0152) -> (-10.0895, 38.3945)
  line L207 (-10.0895, 38.3945) -> (-10.6183, 37.7147)
  line L208 (-10.6183, 37.7147) -> (-11.1015, 37.0016)
  line L209 (-11.1015, 37.0016) -> (-11.9223, 37.5193)
  line L210 (-11.9223, 37.5193) -> (-12.6983, 37.7891)
  line L211 (-12.6983, 37.7891) -> (-13.5587, 37.9123)
  line L212 (-13.5587, 37.9123) -> (-14.4736, 37.9225)
  line L213 (-14.4736, 37.9225) -> (-14.9168, 37.0527)
  line L214 (-14.9168, 37.0527) -> (-14.3707, 36.3185)
  line L215 (-14.3707, 36.3185) -> (-13.7654, 35.6948)
  line L216 (-13.7654, 35.6948) -> (-13.091, 35.2256)
  line L217 (-13.091, 35.2256) -> (-12.1897, 34.8658)
  line L218 (-12.1897, 34.8658) -> (-12.4826, 34.0558)
  line L219 (-12.4826, 34.0558) -> (-12.7218, 33.2284)
extrude "Stage2_Planet_B_Extrude" add sketch "スケッチ1 (15)" along normal blind 12 from surface at 74 separate body makes body 16 in component "Stage2_Planet_Gear_B"
sketch "スケッチ2 (15)" plane through (0, 0, 0) normal (0, 0, 1) x (1, 0, 0) in component "Stage2_Planet_Gear_B"
  circle A0 centre (0, 30) radius 9
extrude "Stage2_Planet_B_Hub_Lower_Extrude" add sketch "スケッチ2 (15)" along normal blind 3 from surface at 71 bodies 16 in component "Stage2_Planet_Gear_B"
sketch "スケッチ3 (14)" plane through (0, 0, 0) normal (0, 0, 1) x (1, 0, 0) in component "Stage2_Planet_Gear_B"
  circle A0 centre (0, 30) radius 9
extrude "Stage2_Planet_B_Hub_Upper_Extrude" add sketch "スケッチ3 (14)" along normal blind 3 from surface at 86 bodies 16 in component "Stage2_Planet_Gear_B"
sketch "スケッチ4 (14)" plane through (0, 0, 0) normal (0, 0, 1) x (1, 0, 0) in component "Stage2_Planet_Gear_B"
  circle A0 centre (0, 30) radius 4.3
extrude "Stage2_Planet_B_Bore_Cut" cut sketch "スケッチ4 (14)" along normal blind 20 from surface at 70 bodies 16 in component "Stage2_Planet_Gear_B"